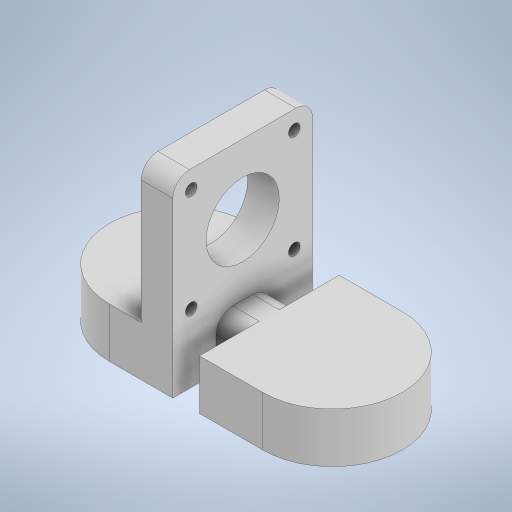
# Autodesk Inventor part: tete
Saved by Autodesk Inventor 2024.1 (Build 281209000, 209)
## iProperties
Created: 2024-04-05
Part Number: tete
Material: Générique
Document SubType Name: Modeling
Designer: chass
Density: 1 g/cm^3
Appearance: Par défaut
Author: chass
Autodesk Inventor part; units mm, degrees
ref_plane "YZ Plane" through (0, 0, 0) normal (1, 0, 0) x (0, 1, 0)
ref_plane "XZ Plane" through (0, 0, 0) normal (0, 1, 0) x (-1, 0, 0)
ref_plane "XY Plane" through (0, 0, 0) normal (0, 0, 1) x (1, 0, 0)
sketch "Esquisse1" plane through (0, 0, 0) normal (1, 0, 0) x (0, 1, 0)
  line L0 (21, 21) -> (-21, 21)
  line L1 (-21, 21) -> (-21, -21)
  line L2 (-21, -21) -> (21, -21)
  line L3 (21, -21) -> (21, 21)
  line L4 (21, 21) -> (-21, -21)
  line L5 (-21, 21) -> (21, -21)
  circle A0 centre (0, 0) radius 11
  line L6 (15.5, 15.5) -> (-15.5, 15.5)
  line L7 (-15.5, 15.5) -> (-15.5, -15.5)
  line L8 (-15.5, -15.5) -> (15.5, -15.5)
  line L9 (15.5, -15.5) -> (15.5, 15.5)
  line L10 (15.5, 15.5) -> (-15.5, -15.5)
  line L11 (-15.5, 15.5) -> (15.5, -15.5)
  circle A1 centre (15.5, 15.5) radius 1.75
  circle A2 centre (-15.5, 15.5) radius 1.75
  line L12 (21, 0) -> (-21, 0)
  circle A3 centre (15.5, -15.5) radius 1.75
  circle A4 centre (-15.5, -15.5) radius 1.75
  point P0 (0, 0)
  point P1 (0, 0)
  dimension "d0" = 42
  dimension "d1" = 22
  dimension "d2" = 31
  dimension "d3" = 3.5
  dimension "d4" = 3.5
  constraints: 26 end point, 6 midpoint, 5 centre point, 4 coincident, 4 parallel, 4 perpendicular, 3 point on line, 2 horizontal, 2 symmetric about line, 2 other
  measures "d0" distance of L2.end L0.start
  measures "d1" diameter of A0
  measures "d2" distance of L8.end L6.start
  measures "d3" diameter of A1
  measures "d4" diameter of A2
extrude "Extrusion1" add sketch "Esquisse1" along normal blind 10 contours L4 A1 L6 A2 L5 L0 | L3 L12 L9 A1 L4 | L5 A2 L7 L12 L1 | L3 L5 A3 L9 L12 | L12 L7 A4 L4 L1 | L2 L4 A4 L8 A3 L5 | L12 A0 L4 A1 L9 | L9 A3 L5 A0 L12 | A1 L4 A0 L5 A2 L6 | L12 A0 L4 A4 L7 | L7 A2 L5 A0 L12 | L8 A4 L4 A0 L5 A3
sketch "Esquisse2" plane through (0, -21, -21) normal (0, -1, 0) x (1, 0, 0)
  point P0 (0, 21)
sketch "Esquisse3" plane through (0, -21, -21) normal (0, -1, 0) x (1, 0, 0)
  line L0 (0, 42) -> (0, 0) projected
  line L1 (0, 42) -> (12, 42)
  line L2 (12, 42) -> (12, 0)
  line L3 (12, 0) -> (0, 0)
  line L4 (0, 0) -> (0, 42)
  point P0 (0, 21)
  dimension "d19" = 12
  constraints: 8 end point, 2 parallel, 1 horizontal, 1 perpendicular
  measures "d19" distance of L2.end L3.end
extrude "Extrusion2" add sketch "Esquisse3" along normal blind 10
sketch "Esquisse4" plane through (10, 0, 0) normal (1, 0, 0) x (0, 0, -1)
  line L0 (21, -31) -> (-21, -31) projected
  line L1 (21, 21) -> (21, -31) projected
  line L2 (-21, -31) -> (21, -31)
  line L3 (21, -31) -> (21, -21)
  line L4 (21, -21) -> (-21, -21)
  line L5 (-21, -21) -> (-21, -31)
  point P0 (0, 0)
  constraints: 8 end point, 2 parallel, 1 horizontal, 1 perpendicular, 1 point on line
extrude "Extrusion3" add sketch "Esquisse4" along normal blind 8
sketch "Esquisse5" plane through (18, 0, 0) normal (1, 0, 0) x (0, 0, -1)
  line L0 (-21, -21) -> (-21, -31) projected
  line L1 (-21, -31) -> (21, -31) projected
  line L2 (-21, -21) -> (21, -21)
  line L3 (21, -21) -> (21, -31)
  line L4 (21, -31) -> (-21, -31)
  line L5 (-21, -31) -> (-21, -21)
  point P0 (0, 0)
  constraints: 8 end point, 2 parallel, 1 horizontal, 1 perpendicular
extrude "Extrusion4" add sketch "Esquisse5" along normal blind 40
sketch "Esquisse9" plane through (10, -21, 21) normal (0, 1, 0) x (1, 0, 0)
  line L0 (0, 0) -> (0, 42) projected
  line L1 (0, 0) -> (48, 0) projected
  line L2 (0, 42) -> (8, 42)
  line L3 (8, 42) -> (8, 0)
  line L4 (8, 0) -> (0, 0)
  line L5 (0, 0) -> (0, 42)
  line L6 (0, 21) -> (8, 21)
  line L7 (0, 29) -> (8, 29)
  line L8 (8, 29) -> (8, 13)
  line L9 (8, 13) -> (0, 13)
  line L10 (0, 13) -> (0, 29)
  point P0 (-10, 21)
  point P1 (0, 13)
  point P2 (8, 29)
  dimension "d24" = 16
  constraints: 18 end point, 4 parallel, 3 point on line, 2 horizontal, 2 midpoint, 2 perpendicular
  measures "d24" distance between parallel lines of L7 L9
extrude "Extrusion7" cut sketch "Esquisse9" against normal blind 10 contours L0 L9 L3 L1 | L0 L2 L3 L7
sketch "Esquisse10" plane through (0, 0, 0) normal (-1, 0, 0) x (0, 0, 1)
  line L0 (21, 21) -> (21, -31) projected
  line L1 (-21, -31) -> (21, -31)
  line L2 (21, -31) -> (21, -21)
  line L3 (21, -21) -> (-21, -21)
  line L4 (-21, -21) -> (-21, -31)
  point P0 (0, 0)
  point P1 (21, -31)
  constraints: 8 end point, 2 parallel, 1 horizontal, 1 perpendicular, 1 point on line
extrude "Extrusion8" add sketch "Esquisse10" along normal blind 30
sketch "Esquisse11" plane through (0, -31, -21) normal (0, -1, 0) x (1, 0, 0)
  line L0 (18, 42) -> (58, 42) projected
  line L1 (18, 0) -> (58, 0) projected
  line L2 (0, 42) -> (-30, 42) projected
  line L3 (10, 29) -> (18, 29) projected
  line L4 (14, 29) -> (14, 13)
  line L5 (18, 13) -> (10, 13) projected
  circle A0 centre (-11, 21) radius 4.05
  circle A1 centre (39, 21) radius 4.05
  point P0 (0, 21)
  point P1 (0, 0)
  point P2 (33, 21)
  point P3 (0, 21)
  point P4 (14, 21)
  dimension "d32" = 8.1
  dimension "d33" = 25
  constraints: 3 midpoint, 2 centre point, 2 end point, 1 coincident, 1 symmetric about line, 1 other
  measures "d32" diameter of A0
  measures "d33" distance of point (14, 21) A0.centre
extrude "Extrusion9" cut sketch "Esquisse11" against normal blind 8
sketch "Esquisse12" plane through (0, -31, -21) normal (0, -1, 0) x (1, 0, 0)
  line L0 (0, 42) -> (-30, 42) projected
  line L1 (-30, 42) -> (10, 42)
  line L2 (10, 42) -> (10, 29)
  line L3 (18, 29) -> (10, 29) projected
  line L4 (18, 42) -> (18, 29) projected
  line L5 (18, 29) -> (18, 42)
  line L6 (18, 42) -> (48, 42)
  line L7 (48, 0) -> (18, 0)
  line L8 (18, 0) -> (18, 13)
  line L9 (18, 13) -> (10, 13)
  line L10 (10, 13) -> (10, 0)
  line L11 (-30, 0) -> (-30, 42)
  line L12 (10, 29) -> (18, 29)
  line L13 (10, 13) -> (18, 13)
  line L14 (0, 0) -> (10, 0) projected
  line L15 (0, 0) -> (10.2767, 0)
  line L16 (0, 0) -> (10, 0)
  line L17 (0, 0) -> (-30, 0) projected
  line L18 (-30, 0) -> (0, 0)
  circle A0 centre (-11, 21) radius 4.05
  circle A1 centre (39, 21) radius 4.05
  line L19 (18, 42) -> (58, 42) projected
  line L20 (48, 42) -> (58, 42)
  line L21 (58, 42) -> (58, 0)
  line L22 (18, 0) -> (58, 0) projected
  line L23 (48, 0) -> (58, 0)
  point P0 (0, 21)
  constraints: 34 end point, 7 point on line, 4 horizontal, 3 perpendicular, 2 centre point, 2 collinear, 1 parallel, 1 vertical
extrude "Extrusion10" add sketch "Esquisse12" along normal blind 5
sketch "Esquisse13" plane through (0, 0, 0) normal (-1, 0, 0) x (0, 0, 1)
  circle A0 centre (-15.5, 15.5) radius 1.75 projected
  circle A1 centre (-15.5, 15.5) radius 1.75
  circle A2 centre (15.5, 15.5) radius 1.75 projected
  circle A3 centre (15.5, 15.5) radius 1.75
  circle A4 centre (15.5, -15.5) radius 1.75 projected
  circle A5 centre (15.5, -15.5) radius 1.75
  circle A6 centre (-15.5, -15.5) radius 1.75 projected
  circle A7 centre (-15.5, -15.5) radius 1.75
  line L0 (-21, -21) -> (21, -21) projected
  line L1 (-21, 21) -> (21, 21)
  line L2 (21, 21) -> (21, -21)
  line L3 (21, -21) -> (-21, -21)
  line L4 (-21, -21) -> (-21, 21)
  circle A8 centre (0, 0) radius 11
  constraints: 8 end point, 5 centre point, 5 coincident, 2 parallel, 1 horizontal, 1 perpendicular
extrude "Extrusion11" cut sketch "Esquisse13" against normal blind 0.5
fillet "Congé5" radius 21 4 edges at (-30, -28.5, 21) (-30, -28.5, -21) (58, -28.5, -21) (58, -28.5, 21)
fillet "Congé6" radius 5 2 edges at (5.25, 21, -21) (5.25, 21, 21)
fillet "Congé7" radius 5 4 edges at (14, -21, -8) (14, -21, 8) (14, -36, 8) (14, -36, -8)
